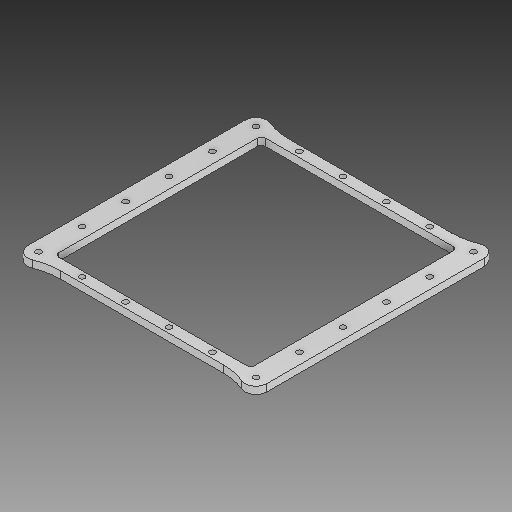
# Autodesk Inventor part: 7525-18-800-002 Battery Mount
Saved by Autodesk Inventor 2022 (Build 260153000, 153)
## iProperties
Created: 2022-01-05
Part Number: 7525-18-800-002 Battery Mount
Material: Aluminum 6061
Document SubType Name: Modeling
Density: 2.7 g/cm^3
Appearance: Aluminum - Dark
Autodesk Inventor part; units mm, degrees
ref_plane "YZ Plane" through (0, 0, 0) normal (1, 0, 0) x (0, 1, 0)
ref_plane "XZ Plane" through (0, 0, 0) normal (0, 1, 0) x (-1, 0, 0)
ref_plane "XY Plane" through (0, 0, 0) normal (0, 0, 1) x (1, 0, 0)
sketch "Battery Flat" plane through (0, 0, 0) normal (0, 0, 1) x (1, 0, 0)
  line L0 (83.566, 88.9) -> (-83.566, 88.9) construction
  line L1 (-83.566, 88.9) -> (-83.566, -88.9) construction
  line L2 (-83.566, -88.9) -> (83.566, -88.9) construction
  line L3 (83.566, -88.9) -> (83.566, 88.9) construction
  line L4 (83.566, 88.9) -> (-83.566, -88.9) construction
  line L5 (-83.566, 88.9) -> (83.566, -88.9) construction
  line L6 (83.566, -88.9) -> (-83.566, -88.9) construction
  line L7 (-83.566, -88.9) -> (-83.566, 88.9) construction
  line L8 (-83.566, 88.9) -> (83.566, 88.9) construction
  line L9 (83.566, 88.9) -> (83.566, -88.9) construction
  point P0 (0, 0)
  dimension "d39" = 167.132
  dimension "d40" = 177.8
  measures "d39" distance of L2.end L1.end
  measures "d40" distance of L1.end L0.end
sketch "Circuit Breaker" plane through (0, 0, 0) normal (0, 0, 1) x (1, 0, 0)
  line L0 (4.1103, 47.4016) -> (-23.8297, 47.4016) construction
  line L1 (-23.8297, 47.4016) -> (-23.8297, -9.7484) construction
  line L2 (-23.8297, -9.7484) -> (4.1103, -9.7484) construction
  line L3 (4.1103, -9.7484) -> (4.1103, 47.4016) construction
  line L4 (4.1103, 47.4016) -> (-23.8297, -9.7484) construction
  line L5 (-23.8297, 47.4016) -> (4.1103, -9.7484) construction
  circle A0 centre (-23.8297, -9.7484) radius 3.429
  circle A1 centre (4.1103, 47.4016) radius 3.429
  line L6 (4.1103, -9.7484) -> (-23.8297, -9.7484) construction
  line L7 (-23.8297, -9.7484) -> (-23.8297, 47.4016) construction
  line L8 (-23.8297, 47.4016) -> (4.1103, 47.4016) construction
  line L9 (4.1103, 47.4016) -> (4.1103, -9.7484) construction
  line L10 (14.2703, 55.6566) -> (-33.9897, 55.6566) construction
  line L11 (-33.9897, 55.6566) -> (-33.9897, -18.0034) construction
  line L12 (-33.9897, -18.0034) -> (14.2703, -18.0034) construction
  line L13 (14.2703, -18.0034) -> (14.2703, 55.6566) construction
  line L14 (14.2703, 55.6566) -> (-33.9897, -18.0034) construction
  line L15 (-33.9897, 55.6566) -> (14.2703, -18.0034) construction
  point P0 (0, 0)
  point P1 (-9.8597, 18.8266)
  dimension "d62" = 27.94
  dimension "d63" = 57.15
  dimension "d64" = 6.858
  dimension "d65" = 6.858
  dimension "d66" = 48.26
  dimension "d67" = 73.66
  measures "d62" distance of L2.end L1.end
  measures "d63" distance of L1.end L0.end
  measures "d64" diameter of A0
  measures "d65" diameter of A1
  measures "d66" distance of L12.end L11.end
  measures "d67" distance of L11.end L10.end
sketch "Sketch1" plane through (0, 0, 0) normal (0, 1, 0) x (-1, 0, 0)
  line L0 (95.25, -95.25) -> (-95.25, -95.25) construction
  line L1 (95.25, -90.4875) -> (-95.25, -90.4875)
  line L2 (-95.25, -100.0125) -> (95.25, -100.0125)
  arc A0 (95.25, -100.0125) -> (95.25, -90.4875) centre (95.25, -95.25) ccw
  arc A1 (-95.25, -90.4875) -> (-95.25, -100.0125) centre (-95.25, -95.25) ccw
  line L3 (95.25, 95.25) -> (-95.25, 95.25) construction
  line L4 (95.25, 100.0125) -> (-95.25, 100.0125)
  line L5 (-95.25, 90.4875) -> (95.25, 90.4875)
  arc A2 (95.25, 90.4875) -> (95.25, 100.0125) centre (95.25, 95.25) ccw
  arc A3 (-95.25, 100.0125) -> (-95.25, 90.4875) centre (-95.25, 95.25) ccw
  line L6 (95.25, -95.25) -> (95.25, 95.25) construction
  line L7 (85.725, -95.25) -> (85.725, 95.25)
  line L8 (104.775, 95.25) -> (104.775, -95.25)
  arc A4 (85.725, -95.25) -> (104.775, -95.25) centre (95.25, -95.25) ccw
  arc A5 (104.775, 95.25) -> (85.725, 95.25) centre (95.25, 95.25) ccw
  line L9 (-95.25, -95.25) -> (-95.25, 95.25) construction
  line L10 (-85.725, -95.25) -> (-85.725, 95.25)
  line L11 (-104.775, 95.25) -> (-104.775, -95.25)
  arc A6 (-104.775, -95.25) -> (-85.725, -95.25) centre (-95.25, -95.25) ccw
  arc A7 (-85.725, 95.25) -> (-104.775, 95.25) centre (-95.25, 95.25) ccw
  circle A8 centre (95.25, -95.25) radius 2.4892
  circle A9 centre (95.25, 95.25) radius 2.4892
  circle A10 centre (57.15, -95.25) radius 2.4892
  circle A11 centre (57.15, 95.25) radius 2.4892
  circle A12 centre (19.05, -95.25) radius 2.4892
  circle A13 centre (19.05, 95.25) radius 2.4892
  circle A14 centre (-19.05, -95.25) radius 2.4892
  circle A15 centre (-19.05, 95.25) radius 2.4892
  circle A16 centre (-57.15, -95.25) radius 2.4892
  circle A17 centre (-57.15, 95.25) radius 2.4892
  circle A18 centre (-95.25, -95.25) radius 2.4892
  circle A19 centre (-95.25, 95.25) radius 2.4892
  circle A20 centre (95.25, 57.15) radius 2.4892
  circle A21 centre (-95.25, 57.15) radius 2.4892
  circle A22 centre (95.25, 19.05) radius 2.4892
  circle A23 centre (-95.25, 19.05) radius 2.4892
  circle A24 centre (95.25, -19.05) radius 2.4892
  circle A25 centre (-95.25, -19.05) radius 2.4892
  circle A26 centre (95.25, -57.15) radius 2.4892
  circle A27 centre (-95.25, -57.15) radius 2.4892
  line L12 (-3.175, 100.0125) -> (-3.175, 150.8125)
  line L13 (-3.175, 150.8125) -> (-79.375, 150.8125)
  line L14 (-79.375, 150.8125) -> (-79.375, 100.0125)
  point P0 (0, 0)
  point P1 (0, 0)
  point P2 (0, -95.25)
  point P3 (0, 95.25)
  point P4 (95.25, 0)
  point P5 (-95.25, 0)
  point P6 (0, 0)
  point P7 (0, 0)
  point P8 (85.725, -90.4875)
  point P9 (-85.725, -90.4875)
  point P10 (-85.725, 90.4875)
  point P11 (85.725, 90.4875)
  point P12 (87.0011, -100.0125)
  point P13 (87.0011, 100.0125)
  point P14 (-87.0011, 100.0125)
  point P15 (-87.0011, -100.0125)
  point P16 (-41.275, 150.8125)
  point P17 (-41.275, 150.8125)
  point P18 (-41.275, 125.4125)
  point P19 (-41.275, 125.4125)
  point P20 (-3.175, 125.4125)
  point P21 (-41.275, 125.4125)
  dimension "d41" = 190.5
  dimension "d42" = 190.5
  dimension "d43" = 9.525
  dimension "d44" = 19.05
  dimension "d45" = 4.9784
  dimension "d48" = 38.1
  dimension "d55" = 38.1
  dimension "d60" = 38.1
  dimension "d68" = 76.2
  dimension "d69" = 50.8
  dimension "d75" = 25.4
  constraints: 38 end point, 28 centre point, 16 point on circle, 16 tangent, 6 midpoint, 5 coincident, 4 parallel, 3 equal radius, 3 horizontal, 3 perpendicular, 3 vertical alignment, 2 concentric, 2 horizontal alignment, 2 point on line, 2 vertical, 42 other
  measures "d41" distance of L0.start L0.end
  measures "d42" distance of L6.start L3.start
  measures "d43" distance between parallel lines of L1 L2
  measures "d44" distance between parallel lines of L8 L7
  measures "d45" diameter of A8
  measures "d48" distance of A8.centre A10.centre
  measures "d55" distance of A9.centre A20.centre
  measures "d60" distance of A26.centre L0.start
  measures "d68" distance of L12.end L13.end
  measures "d69" distance of L12.start L12.end
  measures "d75" distance between parallel lines of L11 L14
extrude "Extrusion1" add sketch "Sketch1" along normal blind 6.35 contours A0 L2 A4 L7 L1 | L1 L7 L5 A2 L4 A5 L8 A4 L2 A0 | L7 A4 L2 A6 L10 L1 | L10 A6 L2 A1 L1 | L1 A1 L2 A6 L11 A7 L4 A3 L5 L10 | L7 A5 L4 A2 L5 | L5 L10 A7 L4 A5 L7 | L5 A3 L4 A7 L10
fillet "Fillet1" radius 50.8 4 edges at (87.0011, 3.175, 100.0125) (-87.0011, 3.175, 100.0125) (-87.0011, 3.175, -100.0125) (87.0011, 3.175, -100.0125)
fillet "Fillet1" radius 3.175 4 edges at (-85.725, 3.175, -90.4875) (85.725, 3.175, -90.4875) (85.725, 3.175, 90.4875) (-85.725, 3.175, 90.4875)
extrude "Extrusion2" [suppressed]
fillet "Fillet2" [suppressed]
sketch "Sketch2" plane through (0, 6.35, 0) normal (0, 1, 0) x (1, 0, 0)
  arc A0 (91.5406, -104.023) -> (71.7571, -100.0125) centre (71.7571, -150.8125) ccw projected
  arc A1 (91.5406, -104.023) -> (104.775, -95.25) centre (95.25, -95.25) ccw projected
  line L0 (104.775, -95.25) -> (104.775, 95.25) projected
  arc A2 (104.775, 95.25) -> (91.5406, 104.023) centre (95.25, 95.25) ccw projected
  arc A3 (71.7571, 100.0125) -> (91.5406, 104.023) centre (71.7571, 150.8125) ccw projected
  line L1 (71.7571, 100.0125) -> (-71.7571, 100.0125) projected
  arc A4 (-91.5406, 104.023) -> (-71.7571, 100.0125) centre (-71.7571, 150.8125) ccw projected
  arc A5 (-91.5406, 104.023) -> (-104.775, 95.25) centre (-95.25, 95.25) ccw projected
  line L2 (-104.775, 95.25) -> (-104.775, -95.25) projected
  arc A6 (-104.775, -95.25) -> (-91.5406, -104.023) centre (-95.25, -95.25) ccw projected
  arc A7 (-71.7571, -100.0125) -> (-91.5406, -104.023) centre (-71.7571, -150.8125) ccw projected
  line L3 (-71.7571, -100.0125) -> (71.7571, -100.0125) projected
  circle A8 centre (-95.25, 95.25) radius 2.4892 projected
  circle A9 centre (-57.15, 95.25) radius 2.4892 projected
  circle A10 centre (-19.05, 95.25) radius 2.4892 projected
  circle A11 centre (19.05, 95.25) radius 2.4892 projected
  circle A12 centre (57.15, 95.25) radius 2.4892 projected
  circle A13 centre (95.25, 95.25) radius 2.4892 projected
  circle A14 centre (-95.25, 57.15) radius 2.4892 projected
  circle A15 centre (-95.25, 19.05) radius 2.4892 projected
  circle A16 centre (-95.25, -19.05) radius 2.4892 projected
  circle A17 centre (-95.25, -57.15) radius 2.4892 projected
  circle A18 centre (-95.25, -95.25) radius 2.4892 projected
  circle A19 centre (-57.15, -95.25) radius 2.4892 projected
  circle A20 centre (-19.05, -95.25) radius 2.4892 projected
  circle A21 centre (19.05, -95.25) radius 2.4892 projected
  circle A22 centre (57.15, -95.25) radius 2.4892 projected
  circle A23 centre (95.25, -95.25) radius 2.4892 projected
  circle A24 centre (95.25, 57.15) radius 2.4892 projected
  circle A25 centre (95.25, -57.15) radius 2.4892 projected
  circle A26 centre (95.25, -19.05) radius 2.4892 projected
  circle A27 centre (95.25, 19.05) radius 2.4892 projected
  line L4 (-82.55, 90.4875) -> (82.55, 90.4875) projected
  arc A28 (85.725, 87.3125) -> (82.55, 90.4875) centre (82.55, 87.3125) ccw projected
  line L5 (85.725, 87.3125) -> (85.725, -87.3125) projected
  arc A29 (82.55, -90.4875) -> (85.725, -87.3125) centre (82.55, -87.3125) ccw projected
  line L6 (82.55, -90.4875) -> (-82.55, -90.4875) projected
  arc A30 (-85.725, -87.3125) -> (-82.55, -90.4875) centre (-82.55, -87.3125) ccw projected
  line L7 (-85.725, -87.3125) -> (-85.725, 87.3125) projected
  arc A31 (-82.55, 90.4875) -> (-85.725, 87.3125) centre (-82.55, 87.3125) ccw projected
  arc A32 (7.9375, -144.4625) -> (9.525, -146.05) centre (9.525, -144.4625) ccw
  line L8 (7.9375, -144.4625) -> (7.9375, -106.3625)
  arc A33 (7.9375, -106.3625) -> (-3.175, -95.25) centre (-3.175, -106.3625) ccw
  line L9 (-3.175, -95.25) -> (-71.7571, -95.25)
  arc A34 (-71.7571, -95.25) -> (-93.3953, -99.6365) centre (-71.7571, -150.8125) ccw
  arc A35 (-100.0125, -95.25) -> (-93.3953, -99.6365) centre (-95.25, -95.25) ccw
  line L10 (-100.0125, -95.25) -> (-100.0125, 95.25)
  arc A36 (-93.3953, 99.6365) -> (-100.0125, 95.25) centre (-95.25, 95.25) ccw
  arc A37 (-93.3953, 99.6365) -> (-71.7571, 95.25) centre (-71.7571, 150.8125) ccw
  line L11 (-71.7571, 95.25) -> (71.7571, 95.25)
  arc A38 (71.7571, 95.25) -> (93.3953, 99.6365) centre (71.7571, 150.8125) ccw
  arc A39 (100.0125, 95.25) -> (93.3953, 99.6365) centre (95.25, 95.25) ccw
  line L12 (100.0125, 95.25) -> (100.0125, -95.25)
  arc A40 (93.3953, -99.6365) -> (100.0125, -95.25) centre (95.25, -95.25) ccw
  arc A41 (93.3953, -99.6365) -> (89.217, -98.0646) centre (71.7571, -150.8125) ccw
  arc A42 (89.217, -98.0646) -> (74.6125, -108.6141) centre (85.725, -108.6141) ccw
  line L13 (74.6125, -108.6141) -> (74.6125, -144.4625)
  arc A43 (73.025, -146.05) -> (74.6125, -144.4625) centre (73.025, -144.4625) ccw
  line L14 (73.025, -146.05) -> (9.525, -146.05)
  arc A44 (3.175, -106.3625) -> (-3.175, -100.0125) centre (-3.175, -106.3625) ccw projected
  line L15 (-3.175, -100.0125) -> (78.6894, -100.0125)
  line L16 (-3.175, -104.775) -> (78.6894, -104.775)
  circle A45 centre (12.7, -111.4425) radius 7.9375
  circle A46 centre (69.85, -139.3825) radius 7.9375
  line L17 (12.7, -111.4425) -> (69.85, -139.3825) construction
  line L18 (11.6541, -113.5818) -> (68.8041, -141.5218)
  line L19 (70.8959, -137.2432) -> (13.7459, -109.3032)
  arc A47 (13.7459, -109.3032) -> (11.6541, -113.5818) centre (12.7, -111.4425) ccw
  arc A48 (68.8041, -141.5218) -> (70.8959, -137.2432) centre (69.85, -139.3825) ccw
  line L20 (2.8572, -144.1945) -> (79.6928, -106.6305) construction
  line L21 (3.9031, -146.3338) -> (80.7387, -108.7697)
  line L22 (78.6469, -104.4912) -> (1.8113, -142.0553)
  arc A49 (1.8113, -142.0553) -> (3.9031, -146.3338) centre (2.8572, -144.1945) ccw
  arc A50 (80.7387, -108.7697) -> (78.6469, -104.4912) centre (79.6928, -106.6305) ccw
  line L23 (41.275, -125.4125) -> (41.275, -104.775) construction
  point P0 (0, 0)
  point P1 (74.6125, -111.7648)
  point P2 (46.6967, -125.4125)
  point P3 (64.0934, -133.9176)
  point P4 (74.6125, -133.0325)
  point P5 (41.275, -122.7619)
  point P6 (74.8457, -106.3496)
  point P7 (75.2967, -104.775)
  point P8 (17.0068, -104.775)
  point P9 (20.5483, -112.6289)
  point P10 (7.9375, -139.0602)
  point P11 (35.8533, -125.4125)
  point P12 (18.4566, -116.9074)
  point P13 (7.9375, -117.7925)
  point P14 (65.5432, -146.05)
  point P15 (62.0017, -138.1961)
  point P16 (41.275, -128.0631)
  point P17 (7.9375, -144.3614)
  dimension "d77" = 4.7625
  dimension "d78" = 15.875
  dimension "d79" = 4.7625
  dimension "d80" = 4.7625
  constraints: 36 end point, 33 point on circle, 18 centre point, 8 tangent, 3 parallel, 2 midpoint, 1 collinear, 1 equal radius, 1 point on line, 1 vertical, 12 other
  measures "d77" distance between parallel lines of L15 L16
  measures "d78" diameter of A45
  measures "d79" diameter of A48
  measures "d80" diameter of A50
extrude "Extrusion3" [suppressed]
fillet "Fillet3" [suppressed]
equation "\"d42\" = d41"
body "Solid1"
